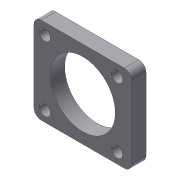
# Autodesk Inventor part: Generic_Pillow_Block
Saved by Autodesk Inventor 2012 (Build 160160000, 160)
## iProperties
Created: 2012-01-24
Part Number: Generic_Pillow_Block
Material: Aluminum-6061
Document SubType Name: Modeling
Designer: JesseK
Density: 2.71 g/cm^3
Mass: 15.632 g
Surface Area: 37.6959 cm^2
Volume: 5.76827 cm^3
Author: JesseK
Autodesk Inventor part; units mm, degrees
ref_plane "YZ Plane" through (0, 0, 0) normal (1, 0, 0) x (0, 1, 0)
ref_plane "XZ Plane" through (0, 0, 0) normal (0, 1, 0) x (-1, 0, 0)
ref_plane "XY Plane" through (0, 0, 0) normal (0, 0, 1) x (1, 0, 0)
sketch "Sketch1" plane through (0, 0, 0) normal (0, 0, 1) x (1, 0, 0)
  circle A0 centre (0, 0) radius 14.2875
  line L0 (-21.4313, 19.05) -> (21.4312, 19.05)
  line L1 (21.4312, 19.05) -> (21.4312, -19.05)
  line L2 (21.4312, -19.05) -> (-21.4312, -19.05)
  line L3 (-21.4312, -19.05) -> (-21.4313, 19.05)
  circle A1 centre (-16.6688, 14.2875) radius 2.4384
  circle A2 centre (15.0812, 14.2875) radius 2.4384
  circle A3 centre (15.0812, -14.2875) radius 2.4384
  circle A4 centre (-16.6687, -14.2875) radius 2.4384
  line L4 (-16.6688, 14.2875) -> (15.0812, 14.2875) construction
  line L5 (15.0812, 14.2875) -> (15.0812, -14.2875) construction
  line L6 (15.0812, -14.2875) -> (-16.6687, -14.2875) construction
  line L7 (-16.6687, -14.2875) -> (-16.6688, 14.2875) construction
  dimension "d0" = 28.575
  dimension "d1" = 42.8625
  dimension "d2" = 38.1
  dimension "d3" = 21.4312
  dimension "d4" = 19.05
  dimension "d5" = 4.8768
  dimension "d6" = 4.7625
  dimension "d7" = 4.7625
  dimension "d8" = 6.35
  dimension "d9" = 4.7625
  dimension "d10" = 31.75
  constraints: 16 end point, 5 centre point, 4 parallel, 3 coincident, 3 equal radius, 2 horizontal, 2 perpendicular
  measures "d0" diameter of A0
  measures "d1" distance of L0.start L0.end
  measures "d2" distance of L2.end L0.start
  measures "d3" distance from line of point (0, 0) L3
  measures "d4" distance from line of point (0, 0) L0
  measures "d5" diameter of A1
  measures "d6" distance between parallel lines of L0 L4
  measures "d7" distance between parallel lines of L2 L6
  measures "d8" distance between parallel lines of L1 L5
  measures "d9" distance between parallel lines of L3 L7
  measures "d10" distance of L5.end L6.end
extrude "Extrusion1" add sketch "Sketch1" along normal blind 6.35
fillet "Fillet1" radius 3.175 4 edges at (21.4312, 19.05, 3.175) (-21.4313, 19.05, 3.175) (21.4312, -19.05, 3.175) (-21.4312, -19.05, 3.175)
body "Solid1"
